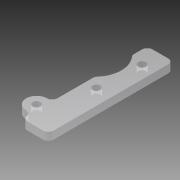
# Autodesk Inventor part: plastic_part_53
Saved by Autodesk Inventor 2013 (Build 170138000, 138)
## iProperties
Shininess: 20.0
Created: 2014-03-15
Part Number: plastic_part_53
Document SubType Name: Modeling
Designer: Noa Izumi
Material: Default
Density: 1 g/cm^3
Density: 0.0
Volumn: 0.0
Area: 0.0
PropertySet Name: Model Information
Control State: 0
Master: False
Checked Out: False
Author: Noa Izumi
Autodesk Inventor part; units mm, degrees
ref_plane "YZ Plane" through (0, 0, 0) normal (1, 0, 0) x (0, 1, 0)
ref_plane "XZ Plane" through (0, 0, 0) normal (0, 1, 0) x (-1, 0, 0)
ref_plane "XY Plane" through (0, 0, 0) normal (0, 0, 1) x (1, 0, 0)
sketch "Sketch1" plane through (0, 0, 0) normal (0, 0, 1) x (1, 0, 0)
  line L0 (0, 0) -> (10, 0)
  line L1 (10, 0) -> (10, 48)
  line L2 (10, 48) -> (0, 48)
  circle A0 centre (-2, 7.5) radius 4
  arc A1 (0, 27.8586) -> (0, 42.1414) centre (-7, 35) ccw
  line L3 (-2, 11.5) -> (0, 11.5)
  line L4 (0, 11.5) -> (0, 3.5)
  line L5 (0, 3.5) -> (-2, 3.5)
  line L6 (-2, 3.5) -> (-2, 11.5)
  line L7 (0, 48) -> (0, 42.1414)
  line L8 (0, 27.8586) -> (0, 0)
  dimension "d90" = 8
  dimension "d0" = 10
  dimension "d1" = 48
  dimension "d88" = 12
  dimension "d89" = 7.5
  dimension "d91" = 20
  dimension "d92" = 13
  constraints: 18 end point, 5 parallel, 2 horizontal, 2 perpendicular, 2 point on circle, 1 centre point, 1 point on line, 1 vertical alignment, 2 other
  measures "d0" distance of L0.start L0.end
  measures "d1" distance of L2.end L0.start
  measures "d88" distance from line of L1 point (-2, 7.5)
  measures "d89" distance from line of L0 point (-2, 7.5)
  measures "d91" diameter of A1
  measures "d92" distance from line of L2 A1.centre
extrude "Extrusion1" add sketch "Sketch1" along normal blind 3
fillet "圓角5" radius 2 8 edges at (0, 0, 1.5) (0, 3.5, 1.5) (0, 11.5, 1.5) (10, 0, 1.5) (0, 27.8586, 1.5) (0, 42.1414, 1.5) (0, 48, 1.5) (10, 48, 1.5)
sketch "草圖9" plane through (0, 0, 3) normal (0, 0, 1) x (1, 0, 0)
  line L0 (2, 48) -> (8, 48) projected
  arc A0 (-2, 11.5) -> (-2, 3.5) centre (-2, 7.5) ccw projected
  line L1 (8, 0) -> (2, 0) projected
  line L2 (10, 46) -> (10, 2) projected
  point P0 (0, 0)
  point P1 (4, 24.5)
  point P2 (5, 41)
  dimension "d95" = 6
  dimension "d96" = 24.5
  dimension "d97" = 7
  dimension "d98" = 5
  constraints: 1 coincident
  measures "d95" distance from line of L2 point (4, 24.5)
  measures "d96" distance from line of L1 point (4, 24.5)
  measures "d97" distance from line of point (5, 41) L0
  measures "d98" distance from line of L2 point (5, 41)
hole "孔5" at (-2, 7.5, 3) at (4, 24.5, 3) at (5, 41, 3) direction (0, 0, -1) diameter 3 end through all
